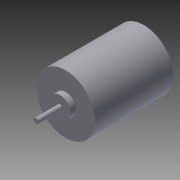
# Autodesk Inventor part: motor kipas
Saved by Autodesk Inventor 2012 (Build 160160000, 160)
## iProperties
Created: 2012-12-20
Part Number: motor kipas
Material: Default
Document SubType Name: Modeling
Designer: Irwan Haryanto
Density: 1 g/cm^3
Author: Irwan Haryanto
Autodesk Inventor part; units mm, degrees
ref_plane "YZ Plane" through (0, 0, 0) normal (1, 0, 0) x (0, 1, 0)
ref_plane "XZ Plane" through (0, 0, 0) normal (0, 1, 0) x (-1, 0, 0)
ref_plane "XY Plane" through (0, 0, 0) normal (0, 0, 1) x (1, 0, 0)
sketch "Sketch1" plane through (0, 0, 0) normal (0, 0, 1) x (1, 0, 0)
  circle A0 centre (0, 0) radius 8.55
  circle A1 centre (0, 0) radius 3.075
  circle A2 centre (0, 0) radius 0.75
  dimension "d0" = 17.1
  dimension "d1" = 6.15
  dimension "d2" = 1.5
  constraints: 3 centre point, 3 coincident
  measures "d0" diameter of A0
  measures "d1" diameter of A1
  measures "d2" diameter of A2
extrude "Extrusion1" add sketch "Sketch1" against normal blind 22.8 contours A0
extrude "Extrusion2" add sketch "Sketch1" along normal blind 1.6 contours A1
extrude "Extrusion3" add sketch "Sketch1" along normal blind 8.6 contours A2
body "Solid1"
